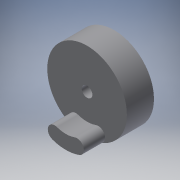
# Autodesk Inventor part: j024 output
Saved by Autodesk Inventor 2016 (Build 200138000, 138)
## iProperties
Created: 2016-09-17
Part Number: j024 output
Material: Generic
Document SubType Name: Modeling
Designer: benja
Density: 1 g/cm^3
Appearance: Default
Author: benja
Autodesk Inventor part; units mm, degrees
ref_plane "YZ Plane" through (0, 0, 0) normal (1, 0, 0) x (0, 1, 0)
ref_plane "XZ Plane" through (0, 0, 0) normal (0, 1, 0) x (-1, 0, 0)
ref_plane "XY Plane" through (0, 0, 0) normal (0, 0, 1) x (1, 0, 0)
sketch "Sketch1" plane through (0, 0, 0) normal (0, 0, 1) x (1, 0, 0)
  circle A0 centre (0, 0) radius 3.9 projected
  circle A1 centre (0, 0) radius 3.75
  dimension "d0" = 7.5
  constraints: 1 centre point, 1 coincident
  measures "d0" diameter of A1
extrude "Extrusion1" add sketch "Sketch1" along normal blind 2.55 contours A1
sketch "Sketch2" plane through (0, 0, 2.55) normal (0, 0, 1) x (1, 0, 0)
  arc A0 (-0.8298, -2.3052) -> (0.8298, -2.3052) centre (0, 0) ccw
  circle A1 centre (0, 0) radius 3.75 projected
  circle A2 centre (0, 0) radius 3.75 projected
  arc A3 (1.2702, -3.5283) -> (0.8298, -2.3052) centre (1.05, -2.9168) ccw
  arc A4 (-0.8298, -2.3052) -> (-1.2702, -3.5283) centre (-1.05, -2.9168) ccw
  line L0 (0, -2.45) -> (0, 0)
  dimension "d3" = 1.3
  dimension "d4" = 3.4
  constraints: 11 point on circle, 4 tangent, 3 centre point, 2 end point, 1 concentric, 1 vertical
  measures "d3" radial gap between concentric circles of A1 A0
extrude "Extrusion2" add sketch "Sketch2" along normal blind 2 contours A0 A3 A1 A4 picked at (0, -3.3001)
sketch "Sketch3" plane through (0, 0, 2.55) normal (0, 0, 1) x (1, 0, 0)
  circle A0 centre (0, 0) radius 0.5
  dimension "d7" = 1
  constraints: 1 centre point, 1 coincident
  measures "d7" diameter of A0
extrude "Extrusion3" cut sketch "Sketch3" against normal blind 2
body "Solid1"
